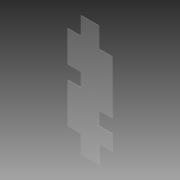
# Autodesk Inventor part: medium tower walls
Saved by Autodesk Inventor 2011 SP1 (Build 150282100, 282)
## iProperties
Created: 2012-01-20
Part Number: medium tower walls
Document SubType Name: Modeling
Designer: Christopher
Density: 1 g/cm^3
Author: Christopher
Autodesk Inventor part; units mm, degrees
ref_plane "YZ Plane" through (0, 0, 0) normal (1, 0, 0) x (0, 1, 0)
ref_plane "XZ Plane" through (0, 0, 0) normal (0, 1, 0) x (-1, 0, 0)
ref_plane "XY Plane" through (0, 0, 0) normal (0, 0, 1) x (1, 0, 0)
sketch "Sketch1" plane through (0, 0, 0) normal (0, 0, 1) x (1, 0, 0)
  line L0 (176.5882, -640.9214) -> (176.5882, 349.6786)
  line L1 (-77.4118, 349.6786) -> (-77.4118, -640.9214)
  line L2 (100.3882, -640.9214) -> (100.3882, -564.7214)
  line L3 (100.3882, -564.7214) -> (176.5882, -564.7214)
  line L4 (176.5882, -475.8214) -> (100.3882, -475.8214)
  line L5 (100.3882, -475.8214) -> (100.3882, -399.6214)
  line L6 (100.3882, -399.6214) -> (176.5882, -399.6214)
  line L7 (176.5882, -399.6214) -> (176.5882, -475.8214)
  line L8 (176.5882, -94.8214) -> (100.3882, -94.8214)
  line L9 (176.5882, 70.2786) -> (176.5882, -94.8214)
  line L10 (-77.4118, 8.6504) -> (-77.4118, 88.2844)
  line L11 (-77.4118, -379.8866) -> (-77.4118, -294.668)
  line L12 (-77.4118, -640.9214) -> (-1.2118, -640.9214)
  line L13 (-1.2118, -640.9214) -> (-1.2118, -564.7214)
  line L14 (-1.2118, -564.7214) -> (-77.4118, -564.7214)
  line L15 (-77.4118, -564.7214) -> (-77.4118, -640.9214)
  line L16 (-77.4118, -259.9214) -> (-1.2118, -259.9214)
  line L17 (-1.2118, -259.9214) -> (-1.2118, -336.1214)
  line L18 (-1.2118, -336.1214) -> (-77.4118, -336.1214)
  line L19 (-77.4118, -336.1214) -> (-77.4118, -259.9214)
  line L20 (-1.2118, -82.1214) -> (-1.2118, 19.4786)
  line L21 (-77.4118, 19.4786) -> (-77.4118, 19.4786)
  line L22 (100.3882, -640.9214) -> (100.3882, -666.3214)
  line L23 (100.3882, -666.3214) -> (-1.2118, -666.3214)
  line L24 (-1.2118, -666.3214) -> (-1.2118, -640.9214)
  line L25 (-1.2118, -82.1214) -> (-77.4118, -82.1214)
  line L26 (100.3882, 19.4786) -> (100.3882, -94.8214)
  line L27 (100.3882, 19.4786) -> (-1.2118, 19.4786)
  point P0 (0, 0)
  point P1 (49.5882, -323.4214)
  point P2 (-64.7118, -437.7214)
  point P3 (-64.7118, -132.9214)
  point P4 (163.8882, -196.4214)
  point P5 (163.8882, -513.9214)
  point P6 (49.5882, -653.6214)
  point P7 (49.5882, 6.7786)
  dimension "d1" = 990.6
  dimension "d2" = 76.2
  dimension "d3" = 76.2
  dimension "d4" = 76.2
  dimension "d5" = 76.2
  dimension "d6" = 88.9
  dimension "d7" = 304.8
  dimension "d14" = 76.2
  dimension "d15" = 76.2
  dimension "d16" = 76.2
  dimension "d17" = 76.2
  dimension "d18" = 63.5
  dimension "d19" = 101.6
  dimension "d20" = 76.2
  dimension "d29" = 12.7
  dimension "d30" = 12.7
  dimension "d31" = 127
  dimension "d32" = 101.6
  dimension "d33" = 12.7
  dimension "d34" = 12.7
  dimension "d35" = 101.6
  dimension "d36" = 38.1
  dimension "d37" = 25.4
  dimension "d38" = 101.6
  dimension "d49" = 101.6
  dimension "d50" = 114.3
  dimension "d51" = 76.2
  dimension "d52" = 76.2
  constraints: 56 end point, 10 parallel, 8 perpendicular, 8 point on line, 4 horizontal
  measures "d1" distance of L1.start L1.end
  measures "d2" distance of L2.start L2.end
  measures "d3" distance of L2.end L3.end
  measures "d4" distance of L4.end L5.end
  measures "d5" distance of L5.end L6.end
  measures "d6" distance between parallel lines of L4 L3
  measures "d7" distance between parallel lines of L8 L6
  measures "d14" distance of L13.end L14.end
  measures "d15" distance of L12.end L13.end
  measures "d16" distance of L16.start L16.end
  measures "d17" distance of L16.end L17.end
  measures "d18" distance between parallel lines of L6 L18
  measures "d19" distance of L20.start L20.end
  measures "d20" distance of L20.end L21.start
  measures "d29" distance from line of L1 point (-64.712, -132.921)
  measures "d30" distance from line of L18 point (49.588, -323.421)
  measures "d31" distance from line of L0 point (49.588, -323.421)
  measures "d32" distance from line of L18 point (-64.712, -437.721)
  measures "d33" distance from line of L1 point (-64.712, -437.721)
  measures "d34" distance from line of L0 point (163.888, -196.421)
  measures "d35" distance from line of L8 point (163.888, -196.421)
  measures "d36" distance from line of L4 point (163.888, -513.921)
  measures "d37" distance of L2.start L22.end
  measures "d38" distance of L22.end L23.end
  measures "d49" distance of L26.start L20.end
  measures "d50" distance of L26.start L8.end
  measures "d51" distance of L20.start L25.end
  measures "d52" distance of L8.start L8.end
extrude "Extrusion1" add sketch "Sketch1" against normal blind 3.175 contours L3 L2 L22 L23 L24 L13 L14 L1 L18 L17 L16 L25 L20 L27 L26 L8 L0 L6 L5 L4
hole "Hole1" at (49.5882, -323.4214, 0) at (-64.7118, -437.7214, 0) at (-64.7118, -132.9214, 0) at (163.8882, -196.4214, 0) at (163.8882, -513.9214, 0) at (49.5882, -653.6214, 0) at (49.5882, 6.7786, 0) direction (0, 0, -1) diameter 6.35 depth 25.4 tip angle 118
body "Solid1"
